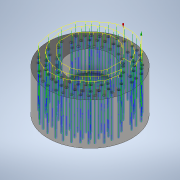
# Autodesk Inventor part: Piston
Saved by Autodesk Inventor 2022 (Build 260153000, 153)
## iProperties
Created: 2021-07-29
Part Number: Piston
Material: Steel, High Strength, Low Alloy
Document SubType Name: Modeling
Designer: WASHINGTON
Density: 7.85 g/cm^3
Appearance: Steel - Polished
Author: WASHINGTON
Autodesk Inventor part; units mm, degrees
ref_plane "YZ Plane" through (0, 0, 0) normal (1, 0, 0) x (0, 1, 0)
ref_plane "XZ Plane" through (0, 0, 0) normal (0, 1, 0) x (-1, 0, 0)
ref_plane "XY Plane" through (0, 0, 0) normal (0, 0, 1) x (1, 0, 0)
sketch "Sketch2" plane through (0, 0, 0) normal (0, 1, 0) x (-1, 0, 0)
  circle A0 centre (0, 0) radius 20
  circle A1 centre (0, 0) radius 10
  dimension "d0" = 40
  dimension "d1" = 20
  constraints: 2 centre point, 2 coincident
  measures "d0" diameter of A0
  measures "d1" diameter of A1
extrude "Extrusion1" add sketch "Sketch2" along normal blind 20
sketch "Sketch3" plane through (0, 0, 0) normal (0, -1, 0) x (1, 0, 0)
  circle A0 centre (0, 0) radius 10
  dimension "d4" = 20
  constraints: 1 centre point, 1 coincident
  measures "d4" diameter of A0
extrude "Extrusion2" add sketch "Sketch3" against normal blind 10
sketch "Sketch4" plane through (0, 20, 0) normal (0, 1, 0) x (1, 0, 0)
  circle A0 centre (0, 0) radius 20 projected
  line L0 (20, 0) -> (-20, 0)
  circle A1 centre (15, 0) radius 0.6
  circle A2 centre (14.0757, 5.1842) radius 0.6
  circle A3 centre (12.5088, 8.2783) radius 0.6
  circle A4 centre (10.7123, 10.4999) radius 0.6
  circle A5 centre (8.7507, 12.183) radius 0.6
  circle A6 centre (6.3855, 13.573) radius 0.6
  circle A7 centre (3.4104, 14.6072) radius 0.6
  circle A8 centre (1.3784, 14.9365) radius 0.6
  circle A9 centre (1.9784, 11.583) radius 0.6
  circle A10 centre (4.766, 10.4999) radius 0.6
  circle A11 centre (6.9855, 8.8783) radius 0.6
  circle A12 centre (8.1507, 7.6783) radius 0.6
  circle A13 centre (10.7123, 5.1842) radius 0.6
  circle A14 centre (11.5777, 3.1207) radius 0.6
  circle A15 centre (1.9784, 18.2579) radius 0.6
  circle A16 centre (4.766, 17.6579) radius 0.6
  circle A17 centre (7.5507, 16.3405) radius 0.6
  circle A18 centre (9.8117, 14.3365) radius 0.6
  circle A19 centre (12.1777, 12.783) radius 0.6
  circle A20 centre (13.4757, 11.0999) radius 0.6
  circle A21 centre (15.6, 8.8783) radius 0.6
  circle A22 centre (16.2, 5.7842) radius 0.6
  circle A23 centre (16.8, 3.1207) radius 0.6
  circle A24 centre (-15, 0) radius 0.6
  circle A25 centre (-14.0757, 5.1842) radius 0.6
  circle A26 centre (-12.5088, 8.2783) radius 0.6
  circle A27 centre (-10.7123, 10.4999) radius 0.6
  circle A28 centre (-8.7507, 12.183) radius 0.6
  circle A29 centre (-6.3855, 13.573) radius 0.6
  circle A30 centre (-3.4104, 14.6072) radius 0.6
  circle A31 centre (-1.3784, 14.9365) radius 0.6
  circle A32 centre (-1.9784, 11.583) radius 0.6
  circle A33 centre (-4.766, 10.4999) radius 0.6
  circle A34 centre (-6.9855, 8.8783) radius 0.6
  circle A35 centre (-8.1507, 7.6783) radius 0.6
  circle A36 centre (-10.7123, 5.1842) radius 0.6
  circle A37 centre (-11.5777, 3.1207) radius 0.6
  circle A38 centre (-1.9784, 18.2579) radius 0.6
  circle A39 centre (-4.766, 17.6579) radius 0.6
  circle A40 centre (-7.5507, 16.3405) radius 0.6
  circle A41 centre (-9.8117, 14.3365) radius 0.6
  circle A42 centre (-12.1777, 12.783) radius 0.6
  circle A43 centre (-13.4757, 11.0999) radius 0.6
  circle A44 centre (-15.6, 8.8783) radius 0.6
  circle A45 centre (-16.8, 3.1207) radius 0.6
  line L1 (20, 0) -> (-20, 0)
  circle A46 centre (15, 0) radius 0.6
  circle A47 centre (14.0757, -5.1842) radius 0.6
  circle A48 centre (12.5088, -8.2783) radius 0.6
  circle A49 centre (10.7123, -10.4999) radius 0.6
  circle A50 centre (8.7507, -12.183) radius 0.6
  circle A51 centre (6.3855, -13.573) radius 0.6
  circle A52 centre (3.4104, -14.6072) radius 0.6
  circle A53 centre (1.3784, -14.9365) radius 0.6
  circle A54 centre (1.9784, -11.583) radius 0.6
  circle A55 centre (4.766, -10.4999) radius 0.6
  circle A56 centre (6.9855, -8.8783) radius 0.6
  circle A57 centre (8.1507, -7.6783) radius 0.6
  circle A58 centre (10.7123, -5.1842) radius 0.6
  circle A59 centre (11.5777, -3.1207) radius 0.6
  circle A60 centre (1.9784, -18.2579) radius 0.6
  circle A61 centre (4.766, -17.6579) radius 0.6
  circle A62 centre (7.5507, -16.3405) radius 0.6
  circle A63 centre (9.8117, -14.3365) radius 0.6
  circle A64 centre (12.1777, -12.783) radius 0.6
  circle A65 centre (13.4757, -11.0999) radius 0.6
  circle A66 centre (15.6, -8.8783) radius 0.6
  circle A67 centre (16.2, -5.7842) radius 0.6
  circle A68 centre (16.8, -3.1207) radius 0.6
  circle A69 centre (-6.9855, -8.8783) radius 0.6
  circle A70 centre (-8.1507, -7.6783) radius 0.6
  circle A71 centre (-15, 0) radius 0.6
  circle A72 centre (-14.0757, -5.1842) radius 0.6
  circle A73 centre (-12.5088, -8.2783) radius 0.6
  circle A74 centre (-10.7123, -5.1842) radius 0.6
  circle A75 centre (-11.5777, -3.1207) radius 0.6
  circle A76 centre (-1.9784, -11.583) radius 0.6
  circle A77 centre (-4.766, -10.4999) radius 0.6
  circle A78 centre (-3.4104, -14.6072) radius 0.6
  circle A79 centre (-1.9784, -18.2579) radius 0.6
  circle A80 centre (-4.766, -17.6579) radius 0.6
  circle A81 centre (-6.3855, -13.573) radius 0.6
  circle A82 centre (-8.7507, -12.183) radius 0.6
  circle A83 centre (-7.5507, -16.3405) radius 0.6
  circle A84 centre (-10.7123, -10.4999) radius 0.6
  circle A85 centre (-12.1777, -12.783) radius 0.6
  circle A86 centre (-9.8117, -14.3365) radius 0.6
  circle A87 centre (-1.3784, -14.9365) radius 0.6
  circle A88 centre (-13.4757, -11.0999) radius 0.6
  circle A89 centre (-15.6, -8.8783) radius 0.6
  circle A90 centre (-16.8, -3.1207) radius 0.6
  point P0 (-16.2, 5.7842)
  point P1 (-16.2, -5.7842)
  dimension "d8" = 1.2
  dimension "d9" = 1.2
  dimension "d10" = 1.2
  dimension "d11" = 1.2
  dimension "d12" = 1.2
  dimension "d13" = 1.2
  dimension "d14" = 1.2
  dimension "d15" = 1.2
  dimension "d16" = 1.2
  dimension "d17" = 1.2
  dimension "d18" = 1.2
  dimension "d19" = 1.2
  dimension "d20" = 1.2
  dimension "d21" = 1.2
  dimension "d22" = 1.2
  dimension "d23" = 1.2
  dimension "d24" = 1.2
  dimension "d25" = 1.2
  dimension "d26" = 1.2
  dimension "d27" = 1.2
  dimension "d28" = 1.2
  dimension "d29" = 1.2
  dimension "d30" = 1.2
  constraints: 90 centre point, 44 symmetric about line, 4 end point, 2 point on circle, 1 collinear, 1 horizontal, 1 point on line, 45 other
  measures "d8" diameter of A1
  measures "d9" diameter of A2
  measures "d10" diameter of A3
  measures "d11" diameter of A4
  measures "d12" diameter of A5
  measures "d13" diameter of A6
  measures "d14" diameter of A7
  measures "d15" diameter of A8
  measures "d16" diameter of A9
  measures "d17" diameter of A10
  measures "d18" diameter of A11
  measures "d19" diameter of A12
  measures "d20" diameter of A13
  measures "d21" diameter of A14
  measures "d22" diameter of A15
  measures "d23" diameter of A16
  measures "d24" diameter of A17
  measures "d25" diameter of A18
  measures "d26" diameter of A19
  measures "d27" diameter of A20
  measures "d28" diameter of A21
  measures "d29" diameter of A22
  measures "d30" diameter of A23
hole "Hole1" at (-9.8117, 20, -14.3365) at (-8.7507, 20, -12.183) at (-6.9855, 20, -8.8783) at (-10.7123, 20, -10.4999) at (-12.1777, 20, -12.783) at (-13.4757, 20, -11.0999) at (-12.5088, 20, -8.2783) at (-8.1507, 20, -7.6783) at (-10.7123, 20, -5.1842) at (-15.6, 20, -8.8783) at (-14.0757, 20, -5.1842) at (-11.5777, 20, -3.1207) at (-16.8, 20, -3.1207) at (-15, 20, 0) at (-16.8, 20, 3.1207) at (-14.0757, 20, 5.1842) at (-11.5777, 20, 3.1207) at (-10.7123, 20, 5.1842) at (-12.5088, 20, 8.2783) at (-15.6, 20, 8.8783) at (-13.4757, 20, 11.0999) at (-10.7123, 20, 10.4999) at (-8.1507, 20, 7.6783) at (-6.9855, 20, 8.8783) at (-8.7507, 20, 12.183) at (-9.8117, 20, 14.3365) at (-7.5507, 20, 16.3405) at (-6.3855, 20, 13.573) at (-4.766, 20, 10.4999) at (-1.9784, 20, 11.583) at (-3.4104, 20, 14.6072) at (-4.766, 20, 17.6579) at (-1.9784, 20, 18.2579) at (-1.3784, 20, 14.9365) at (1.3784, 20, 14.9365) at (1.9784, 20, 18.2579) at (4.766, 20, 17.6579) at (3.4104, 20, 14.6072) at (1.9784, 20, 11.583) at (4.766, 20, 10.4999) at (6.3855, 20, 13.573) at (7.5507, 20, 16.3405) at (9.8117, 20, 14.3365) at (8.7507, 20, 12.183) at (6.9855, 20, 8.8783) at (8.1507, 20, 7.6783) at (10.7123, 20, 10.4999) at (12.1777, 20, 12.783) at (12.5088, 20, 8.2783) at (10.7123, 20, 5.1842) direction (0, -1, 0) diameter 1.2 end through all and at (15.6, 20, 8.8783) (13.4757, 20, 11.0999) (16.2, 20, 5.7842) (14.0757, 20, 5.1842) (11.5777, 20, 3.1207) (16.8, 20, 3.1207) (16.8, 20, -3.1207) (14.0757, 20, -5.1842) (-6.3855, 20, -13.573) (-7.5507, 20, -16.3405) (-4.766, 20, -17.6579) (-3.4104, 20, -14.6072) (-4.766, 20, -10.4999)
hole "Hole2" at (-1.9784, 20, -18.2579) at (-1.9784, 20, -11.583) at (1.9784, 20, -18.2579) at (6.3855, 20, -13.573) at (7.5507, 20, -16.3405) at (9.8117, 20, -14.3365) at (8.7507, 20, -12.183) at (15, 20, 0) at (3.4104, 20, -14.6072) at (1.9784, 20, -11.583) at (12.5088, 20, -8.2783) at (10.7123, 20, -5.1842) at (13.4757, 20, -11.0999) at (12.1777, 20, -12.783) at (10.7123, 20, -10.4999) at (6.9855, 20, -8.8783) at (8.1507, 20, -7.6783) at (4.766, 20, -10.4999) at (4.766, 20, -17.6579) at (-1.3784, 20, -14.9365) at (15.6, 20, -8.8783) at (16.2, 20, -5.7842) at (11.5777, 20, -3.1207) at (16.8, 20, -3.1207) at (14.0757, 20, -5.1842) direction (0, -1, 0) diameter 1.2 end through all
equation "\"d31\" = d16"
equation "\"d38\" = d9"
body "Solid1"
